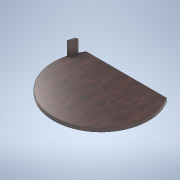
# Autodesk Inventor part: Nest-ver3-1111-2021
Saved by Autodesk Inventor 2021 (Build 250183000, 183)
## iProperties
Created: 2021-03-02
Part Number: Nest-ver3-1111-2021
Material: Generic
Document SubType Name: Modeling
Designer: CMurray
Density: 1 g/cm^3
Appearance: White Oak - Wild Berries
Author: CMurray
Autodesk Inventor part; units mm, degrees
ref_plane "YZ Plane" through (0, 0, 0) normal (1, 0, 0) x (0, 1, 0)
ref_plane "XZ Plane" through (0, 0, 0) normal (0, 1, 0) x (-1, 0, 0)
ref_plane "XY Plane" through (0, 0, 0) normal (0, 0, 1) x (1, 0, 0)
sketch "Sketch2" plane through (0, 0, 0) normal (0, 1, 0) x (-1, 0, 0)
  arc A0 (762, -479.9355) -> (-762, -479.9355) centre (0, 0) ccw
  line L0 (900.5455, 0) -> (762, 0)
  line L1 (762, -479.9355) -> (-762, -479.9355)
  dimension "d8" = 1524
  constraints: 4 end point, 3 point on circle, 1 centre point, 1 coincident, 1 horizontal
  measures "d8" distance of L1.start L1.end
extrude "Extrusion1" add sketch "Sketch2" along normal blind 63.5
sketch "Sketch4" plane through (0, 63.5, 0) normal (0, 1, 0) x (1, 0, 0)
  arc A0 (-762, 479.9355) -> (762, 479.9355) centre (0, 0) ccw
  line L0 (762, 479.9355) -> (-762, 479.9355) projected
  arc A1 (-762, 479.9355) -> (762, 479.9355) centre (0, 0) ccw projected
  line L1 (-762, 479.9355) -> (762, 479.9355)
  line L2 (-790.3185, 352.9355) -> (-828.5038, 352.9355)
  line L3 (-790.3185, 352.9355) -> (-790.3185, 225.9355)
  line L4 (-790.3185, 225.9355) -> (-871.7427, 225.9355)
  dimension "d15" = 127
  constraints: 8 end point, 4 point on circle, 2 horizontal, 1 centre point, 1 coincident, 1 perpendicular, 1 vertical
  measures "d15" distance of L2.start L3.end
extrude "Extrusion4" add sketch "Sketch4" along normal blind 254 contours L2 L3 L4 A0
sketch "Sketch8" plane through (0, 63.5, 0) normal (0, 1, 0) x (1, 0, 0)
  arc A0 (-762, 479.9355) -> (762, 479.9355) centre (0, 0) ccw
  line L0 (762, 479.9355) -> (-762, 479.9355) projected
  line L1 (762, 479.9355) -> (-762, 479.9355)
  arc A1 (-733.4235, 429.1355) -> (733.4235, 429.1355) centre (0, 0) ccw
  line L2 (-733.4235, 429.1355) -> (733.4235, 429.1355)
  dimension "d39" = 50.8
  constraints: 4 end point, 4 point on circle, 2 centre point, 1 coincident, 1 collinear, 1 other
  measures "d39" radial gap between concentric circles of A0 A1
extrude "Extrusion9" cut sketch "Sketch8" along normal blind 381 contours L2 A1
body "Solid1"
